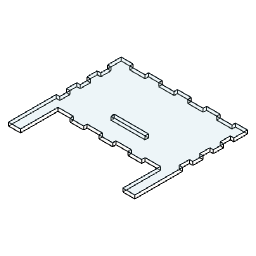
case_2_2mm (Autodesk Fusion 360 design; units mm, degrees)
Autodesk Fusion 360 part; units mm, degrees
sketch "スケッチ1" plane through (0, 0, 0) normal (0, 0, 1) x (1, 0, 0)
  line L0 (0, 0) -> (74, 0)
  line L1 (74, 0) -> (74, 46)
  line L2 (74, 46) -> (0, 46)
  line L3 (0, 46) -> (0, 0)
  dimension "d1" = 46
  dimension "d2" = 74
  constraint horizontal L0
  constraint vertical L1
  constraint horizontal L2
  constraint vertical L3
  constraint coincident L0.start L3.end
  measures "d1" distance of L0.start L2.end
  measures "d2" distance of L0.start L0.end
extrude "押し出し1" add sketch "スケッチ1" along normal blind 2
sketch "スケッチ2" plane through (0, 0, 2) normal (0, 0, 1) x (-1, 0, 0)
  line L0 (0, -46) -> (0, 0)
  line L1 (0, 0) -> (-74, 0)
  line L2 (-74, 0) -> (-74, -46)
  line L3 (-74, -46) -> (0, -46)
  line L4 (-27, -13) -> (-47, -13)
  line L5 (-47, -13) -> (-47, -15)
  line L6 (-47, -15) -> (-27, -15)
  line L7 (-27, -15) -> (-27, -13)
  dimension "d5" = 2
  dimension "d6" = 20
  dimension "d7" = 13
  dimension "d8" = 27
  constraint horizontal L4
  constraint vertical L5
  constraint horizontal L6
  constraint vertical L7
  measures "d5" distance of L4.end L5.end
  measures "d6" distance of L4.start L4.end
  measures "d7" distance of L1 L4
  measures "d8" distance of L2 L5
extrude "押し出し2" cut sketch "スケッチ2" against normal blind 2 contours L4 L5 L6 L7
sketch "スケッチ3" plane through (0, 0, 2) normal (0, 0, 1) x (-1, 0, 0)
  line L0 (-47, -13) -> (-27, -13)
  line L1 (-27, -13) -> (-27, -15)
  line L2 (-27, -15) -> (-47, -15)
  line L3 (-47, -15) -> (-47, -13)
  line L4 (0, -46) -> (0, 0)
  line L5 (0, 0) -> (-74, 0)
  line L6 (-74, 0) -> (-74, -46)
  line L7 (-74, -46) -> (0, -46)
  line L8 (-67, -46) -> (-58, -46)
  line L9 (-58, -46) -> (-58, -44)
  line L10 (-58, -44) -> (-67, -44)
  line L11 (-67, -44) -> (-67, -46)
  line L12 (-50, -46) -> (-41, -46)
  line L13 (-50, -44) -> (-50, -46)
  line L14 (-41, -44) -> (-50, -44)
  line L15 (-41, -46) -> (-41, -44)
  line L16 (-33, -46) -> (-24, -46)
  line L17 (-33, -44) -> (-33, -46)
  line L18 (-24, -44) -> (-33, -44)
  line L19 (-24, -46) -> (-24, -44)
  line L20 (-16, -46) -> (-7, -46)
  line L21 (-16, -44) -> (-16, -46)
  line L22 (-7, -44) -> (-16, -44)
  line L23 (-7, -46) -> (-7, -44)
  line L24 (-24, 0) -> (-33, 0)
  line L25 (-33, 0) -> (-33, -2)
  line L26 (-58, 0) -> (-67, 0)
  line L27 (-50, 0) -> (-50, -2)
  line L28 (-50, -2) -> (-41, -2)
  line L29 (-7, -2) -> (-7, 0)
  line L30 (-7, 0) -> (-16, 0)
  line L31 (-16, 0) -> (-16, -2)
  line L32 (-33, -2) -> (-24, -2)
  line L33 (-67, 0) -> (-67, -2)
  line L34 (-41, -2) -> (-41, 0)
  line L35 (-16, -2) -> (-7, -2)
  line L36 (-24, -2) -> (-24, 0)
  line L37 (-41, 0) -> (-50, 0)
  line L38 (-67, -2) -> (-58, -2)
  line L39 (-58, -2) -> (-58, 0)
  line L40 (0, -38) -> (-2, -38)
  line L41 (-2, -38) -> (-2, -32)
  line L42 (-2, -32) -> (0, -32)
  line L43 (0, -32) -> (0, -38)
  line L44 (-2, -20) -> (0, -20)
  line L45 (-2, -26) -> (-2, -20)
  line L46 (0, -26) -> (-2, -26)
  line L47 (0, -20) -> (0, -26)
  line L48 (-2, -8) -> (0, -8)
  line L49 (-2, -14) -> (-2, -8)
  line L50 (0, -14) -> (-2, -14)
  line L51 (0, -8) -> (0, -14)
  line L52 (-74, -20) -> (-72, -20)
  line L53 (-72, -8) -> (-72, -14)
  line L54 (-74, -8) -> (-72, -8)
  line L55 (-72, -14) -> (-74, -14)
  line L56 (-74, -38) -> (-74, -32)
  line L57 (-72, -32) -> (-72, -38)
  line L58 (-72, -26) -> (-74, -26)
  line L59 (-74, -32) -> (-72, -32)
  line L60 (-74, -14) -> (-74, -8)
  line L61 (-72, -20) -> (-72, -26)
  line L62 (-74, -26) -> (-74, -20)
  line L63 (-72, -38) -> (-74, -38)
  dimension "d11" = 9
  dimension "d12" = 2
  dimension "d13" = 7
  dimension "d16" = 17
  dimension "d17" = 0
  dimension "d20" = 0
  dimension "d21" = 44
  dimension "d22" = 6
  dimension "d23" = 2
  dimension "d24" = 8
  dimension "d27" = 0
  dimension "d28" = 12
  dimension "d31" = -72
  dimension "d32" = 0
  constraint horizontal L8
  constraint vertical L9
  constraint horizontal L10
  constraint vertical L11
  constraint coincident L7 L8.start
  constraint horizontal L40
  constraint vertical L41
  constraint horizontal L42
  constraint vertical L43
  constraint coincident L4 L40.start
  measures "d11" distance of L8.start L8.end
  measures "d12" distance of L8.start L10.end
  measures "d13" distance of L6 L11
  measures "d22" distance of L40.start L42.end
  measures "d23" distance of L40.start L40.end
  measures "d24" distance of L7 L40
extrude "押し出し3" cut sketch "スケッチ3" against normal blind 2 contours L4 L40 L41 L42 L43 | L7 L20 L21 L22 L23 | L4 L44 L45 L46 L47 | L7 L16 L17 L18 L19 | L4 L48 L49 L50 L51 | L7 L12 L13 L14 L15 | L7 L8 L9 L10 L11 | L5 L29 L30 L31 L35 | L5 L24 L25 L32 L36 | L6 L56 L57 L59 L63 | L5 L27 L28 L34 L37 | L6 L52 L58 L61 L62 | L5 L26 L33 L38 L39 | L6 L53 L54 L55 L60
sketch "スケッチ4" plane through (0, 0, 2) normal (0, 0, 1) x (-1, 0, 0)
  line L0 (-50, -2) -> (-50, 0)
  line L1 (-50, 0) -> (-58, 0)
  line L2 (-58, 0) -> (-58, -2)
  line L3 (-58, -2) -> (-67, -2)
  line L4 (-67, -2) -> (-67, 0)
  line L5 (-67, 0) -> (-74, 0)
  line L6 (-74, 0) -> (-74, -8)
  line L7 (-74, -8) -> (-72, -8)
  line L8 (-72, -8) -> (-72, -14)
  line L9 (-72, -14) -> (-74, -14)
  line L10 (-74, -14) -> (-74, -20)
  line L11 (-74, -20) -> (-72, -20)
  line L12 (-72, -20) -> (-72, -26)
  line L13 (-72, -26) -> (-74, -26)
  line L14 (-74, -26) -> (-74, -32)
  line L15 (-74, -32) -> (-72, -32)
  line L16 (-72, -32) -> (-72, -38)
  line L17 (-72, -38) -> (-74, -38)
  line L18 (-74, -38) -> (-74, -46)
  line L19 (-74, -46) -> (-67, -46)
  line L20 (-67, -46) -> (-67, -44)
  line L21 (-67, -44) -> (-58, -44)
  line L22 (-58, -44) -> (-58, -46)
  line L23 (-58, -46) -> (-50, -46)
  line L24 (-50, -46) -> (-50, -44)
  line L25 (-50, -44) -> (-41, -44)
  line L26 (-41, -44) -> (-41, -46)
  line L27 (-41, -46) -> (-33, -46)
  line L28 (-33, -46) -> (-33, -44)
  line L29 (-33, -44) -> (-24, -44)
  line L30 (-24, -44) -> (-24, -46)
  line L31 (-24, -46) -> (-16, -46)
  line L32 (-16, -46) -> (-16, -44)
  line L33 (-16, -44) -> (-7, -44)
  line L34 (-7, -44) -> (-7, -46)
  line L35 (-7, -46) -> (0, -46)
  line L36 (0, -46) -> (0, -38)
  line L37 (0, -38) -> (-2, -38)
  line L38 (-2, -38) -> (-2, -32)
  line L39 (-2, -32) -> (0, -32)
  line L40 (0, -32) -> (0, -26)
  line L41 (0, -26) -> (-2, -26)
  line L42 (-2, -26) -> (-2, -20)
  line L43 (-2, -20) -> (0, -20)
  line L44 (0, -20) -> (0, -14)
  line L45 (0, -14) -> (-2, -14)
  line L46 (-2, -14) -> (-2, -8)
  line L47 (-2, -8) -> (0, -8)
  line L48 (0, -8) -> (0, 0)
  line L49 (0, 0) -> (-7, 0)
  line L50 (-7, 0) -> (-7, -2)
  line L51 (-7, -2) -> (-16, -2)
  line L52 (-16, -2) -> (-16, 0)
  line L53 (-16, 0) -> (-24, 0)
  line L54 (-24, 0) -> (-24, -2)
  line L55 (-24, -2) -> (-33, -2)
  line L56 (-33, -2) -> (-33, 0)
  line L57 (-33, 0) -> (-41, 0)
  line L58 (-41, 0) -> (-41, -2)
  line L59 (-41, -2) -> (-50, -2)
  line L60 (-47, -13) -> (-27, -13)
  line L61 (-27, -13) -> (-27, -15)
  line L62 (-27, -15) -> (-47, -15)
  line L63 (-47, -15) -> (-47, -13)
  line L64 (0, 0) -> (0, 20)
  line L65 (0, 20) -> (-7, 20)
  line L66 (-7, 20) -> (-7, 0)
  line L67 (-74, 0) -> (-74, 20)
  line L68 (-74, 20) -> (-67, 20)
  line L69 (-67, 20) -> (-67, 0)
  constraint vertical L64
  constraint horizontal L65
  constraint vertical L66
  constraint coincident L49.end L50.start
  constraint vertical L67
  constraint horizontal L68
  constraint vertical L69
  constraint coincident L4.end L5.start
extrude "押し出し4" add sketch "スケッチ4" against normal blind 2 contours L5 L67 L68 L69 | L49 L64 L65 L66
sketch "スケッチ5" plane through (0, 0, 2) normal (0, 0, 1) x (-1, 0, 0)
  line L0 (-50, -2) -> (-50, 0)
  line L1 (-50, 0) -> (-58, 0)
  line L2 (-58, 0) -> (-58, -2)
  line L3 (-58, -2) -> (-67, -2)
  line L4 (-67, -2) -> (-67, 20)
  line L5 (-67, 20) -> (-74, 20)
  line L6 (-74, 20) -> (-74, -8)
  line L7 (-74, -8) -> (-72, -8)
  line L8 (-72, -8) -> (-72, -14)
  line L9 (-72, -14) -> (-74, -14)
  line L10 (-74, -14) -> (-74, -20)
  line L11 (-74, -20) -> (-72, -20)
  line L12 (-72, -20) -> (-72, -26)
  line L13 (-72, -26) -> (-74, -26)
  line L14 (-74, -26) -> (-74, -32)
  line L15 (-74, -32) -> (-72, -32)
  line L16 (-72, -32) -> (-72, -38)
  line L17 (-72, -38) -> (-74, -38)
  line L18 (-74, -38) -> (-74, -46)
  line L19 (-74, -46) -> (-67, -46)
  line L20 (-67, -46) -> (-67, -44)
  line L21 (-67, -44) -> (-58, -44)
  line L22 (-58, -44) -> (-58, -46)
  line L23 (-58, -46) -> (-50, -46)
  line L24 (-50, -46) -> (-50, -44)
  line L25 (-50, -44) -> (-41, -44)
  line L26 (-41, -44) -> (-41, -46)
  line L27 (-41, -46) -> (-33, -46)
  line L28 (-33, -46) -> (-33, -44)
  line L29 (-33, -44) -> (-24, -44)
  line L30 (-24, -44) -> (-24, -46)
  line L31 (-24, -46) -> (-16, -46)
  line L32 (-16, -46) -> (-16, -44)
  line L33 (-16, -44) -> (-7, -44)
  line L34 (-7, -44) -> (-7, -46)
  line L35 (-7, -46) -> (0, -46)
  line L36 (0, -46) -> (0, -38)
  line L37 (0, -38) -> (-2, -38)
  line L38 (-2, -38) -> (-2, -32)
  line L39 (-2, -32) -> (0, -32)
  line L40 (0, -32) -> (0, -26)
  line L41 (0, -26) -> (-2, -26)
  line L42 (-2, -26) -> (-2, -20)
  line L43 (-2, -20) -> (0, -20)
  line L44 (0, -20) -> (0, -14)
  line L45 (0, -14) -> (-2, -14)
  line L46 (-2, -14) -> (-2, -8)
  line L47 (-2, -8) -> (0, -8)
  line L48 (0, -8) -> (0, 20)
  line L49 (0, 20) -> (-7, 20)
  line L50 (-7, 20) -> (-7, -2)
  line L51 (-7, -2) -> (-16, -2)
  line L52 (-16, -2) -> (-16, 0)
  line L53 (-16, 0) -> (-24, 0)
  line L54 (-24, 0) -> (-24, -2)
  line L55 (-24, -2) -> (-33, -2)
  line L56 (-33, -2) -> (-33, 0)
  line L57 (-33, 0) -> (-41, 0)
  line L58 (-41, 0) -> (-41, -2)
  line L59 (-41, -2) -> (-50, -2)
  line L60 (-47, -13) -> (-27, -13)
  line L61 (-27, -13) -> (-27, -15)
  line L62 (-27, -15) -> (-47, -15)
  line L63 (-47, -15) -> (-47, -13)
